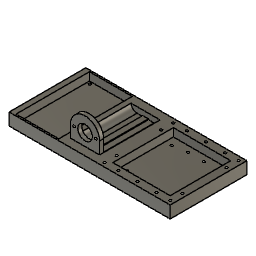
Base Péndulo v4 (Autodesk Fusion 360 design; units mm, degrees)
Autodesk Fusion 360 part; units mm, degrees
note: some values were not read from the file. Set by a fixed rule: which sketch regions a step uses.
sketch "Boceto1" plane through (0, 0, 0) normal (0, 0, 1) x (1, 0, 0)
  line L0 (0, 0) -> (0, 75)
  line L1 (0, 75) -> (71, 75)
  line L2 (71, 75) -> (71, 0)
  line L3 (71, 0) -> (0, 0)
  line L4 (71, 75) -> (81, 75)
  line L5 (81, 75) -> (81, 85)
  line L6 (81, 85) -> (-10, 85)
  line L7 (-10, 85) -> (-10, -10)
  line L8 (-10, -10) -> (81, -10)
  line L9 (81, -10) -> (81, 75)
  dimension "d1" = 75
  dimension "d2" = 71
  dimension "d3" = 10
  constraint coincident L0.start L3.end
  constraint vertical L0
  constraint perpendicular L0 L1
  constraint perpendicular L1 L2
  constraint perpendicular L0 L3
  constraint perpendicular L2 L4
  constraint perpendicular L4 L5
  constraint perpendicular L5 L6
  constraint perpendicular L6 L7
  constraint perpendicular L0 L8
  constraint perpendicular L4 L9
  measures "d1" distance of L0.start L0.end
  measures "d2" distance of L0.end L1.end
  measures "d3" distance of L1.end L4.end
extrude "Extruir1" add sketch "Boceto1" against normal blind 5 contours L0 L1 L2 L3 | L5 L6 L7 L8 L9 makes body 1
extrude "Extruir2" add sketch "Boceto1" along normal blind 10 bodies 1
sketch "Boceto2" plane through (0, 0, 0) normal (0, 0, 1) x (-1, 0, 0)
  line L0 (-71, -75) -> (0, -75)
  line L1 (0, -75) -> (0, 0)
  line L2 (0, 0) -> (-71, 0)
  line L3 (-71, 0) -> (-71, -75)
  line L4 (-35.5, -75) -> (-70.5, -75)
  line L5 (-35.5, -75) -> (-0.5, -75)
  line L6 (-0.5, -75) -> (-0.5, -55)
  line L7 (-0.5, -55) -> (-70.5, -55)
  line L8 (-70.5, -55) -> (-70.5, -75)
  line L9 (-0.5, -55) -> (-15.5, -55)
  line L10 (-15.5, -55) -> (-15.5, -75)
  line L11 (-70.5, -55) -> (-55.5, -55)
  line L12 (-55.5, -55) -> (-55.5, -75)
  line L13 (-15.5, -55) -> (-0.5, -75)
  line L14 (-55.5, -55) -> (-70.5, -75)
  line L15 (-15.5, -75) -> (-15.5, -60)
  line L16 (-15.5, -60) -> (-55.5, -60)
  line L17 (-35.5, -60) -> (-35.5, -75)
  line L18 (-35.5, -67.5) -> (-15.5, -67.5)
  line L19 (-35.5, -67.5) -> (-55.5, -67.5)
  circle A0 centre (-25.5, -67.5) radius 1.5
  circle A1 centre (-45.5, -67.5) radius 1.5
  circle A2 centre (-8, -65) radius 1.5
  circle A3 centre (-63, -65) radius 1.5
  dimension "d8" = 35
  dimension "d9" = 35
  dimension "d10" = 20
  dimension "d11" = 15
  dimension "d12" = 20
  dimension "d13" = 15
  dimension "d14" = 20
  dimension "d15" = 15
  dimension "d16" = 3
  dimension "d17" = 3
  dimension "d18" = 3
  dimension "d19" = 3
  constraint midpoint L0 L4.start
  constraint parallel L0 L4
  constraint parallel L0 L5
  constraint perpendicular L5 L6
  constraint perpendicular L3 L7
  constraint perpendicular L4 L8
  constraint perpendicular L6 L9
  constraint perpendicular L5 L10
  constraint perpendicular L8 L11
  constraint perpendicular L4 L12
  constraint perpendicular L5 L15
  constraint coincident L12 L16.end
  constraint perpendicular L12 L16
  constraint midpoint L16 L17.start
  constraint midpoint L17 L18.start
  constraint midpoint L15 L18.end
  constraint coincident L12 L19.end
  constraint perpendicular L12 L19
  constraint midpoint L18 A0.centre
  constraint midpoint L19 A1.centre
  constraint midpoint L13 A2.centre
  constraint midpoint L14 A3.centre
  measures "d8" distance of L4.start L4.end
  measures "d9" distance of L4.start L5.end
  measures "d10" distance of L5.end L6.end
  measures "d11" distance of L6.end L9.end
  measures "d12" distance of L9.end L10.end
  measures "d13" distance of L7.end L11.end
  measures "d14" distance of L11.end L12.end
  measures "d15" distance of L10.end L15.end
  measures "d16" diameter of A0
  measures "d17" diameter of A1
  measures "d18" diameter of A2
  measures "d19" diameter of A3
extrude "Extruir3" cut sketch "Boceto2" against normal up to surface (5 mm away) contours L14 A3 | L14 A3 | L19 A1 | L19 A1 | L18 A0 | L18 A0 | L13 A2 | L13 A2 bodies 1
sketch "Boceto3" plane through (0, 0, 10) normal (0, 0, 1) x (-1, 0, 0)
  line L0 (-71, -75) -> (-71, 0)
  line L1 (-71, 0) -> (0, 0)
  line L2 (0, 0) -> (0, -75)
  line L3 (0, -75) -> (-71, -75)
  line L4 (-81, 10) -> (-81, -85)
  line L5 (-81, -85) -> (10, -85)
  line L6 (10, -85) -> (10, 10)
  line L7 (10, 10) -> (-81, 10)
  line L8 (-71, -75) -> (-71, -60)
  line L9 (-71, -60) -> (-81, -60)
  line L10 (-81, -60) -> (-81, -85)
  line L11 (-81, -85) -> (10, -85)
  line L12 (0, -75) -> (0, -60)
  line L13 (0, -60) -> (10, -60)
  line L14 (10, -60) -> (10, -85)
  line L15 (0, -75) -> (-71, -75)
  line L16 (0, -75) -> (10, -75)
  line L17 (0, -75) -> (0, -85)
  line L18 (-71, -75) -> (-71, -85)
  line L19 (-71, -75) -> (-81, -75)
  circle A0 centre (5, -80) radius 1.5
  circle A1 centre (-76, -80) radius 1.5
  line L20 (10, -60) -> (0, -70)
  circle A2 centre (5, -65) radius 1.5
  line L21 (-81, -60) -> (-71, -70)
  circle A3 centre (-76, -65) radius 1.5
  line L22 (0, -85) -> (-23.6667, -85)
  line L23 (-71, -85) -> (-47.3333, -85)
  line L24 (-47.3333, -85) -> (-47.3333, -75)
  line L25 (-23.6667, -85) -> (-23.6667, -75)
  line L26 (-23.6667, -85) -> (0, -75)
  line L27 (-23.6667, -85) -> (-47.3333, -75)
  line L28 (-47.3333, -75) -> (-71, -85)
  circle A4 centre (-11.8333, -80) radius 1.5
  circle A5 centre (-35.5, -80) radius 1.5
  circle A6 centre (-59.1667, -80) radius 1.5
  dimension "d22" = 15
  dimension "d23" = 15
  dimension "d24" = 3
  dimension "d25" = 3
  dimension "d26" = 3
  dimension "d27" = 3
  dimension "d28" = 23.6667
  dimension "d29" = 23.6667
  dimension "d30" = 3
  dimension "d31" = 3
  dimension "d32" = 3
  constraint coincident L0.start L3.end
  constraint perpendicular L3 L8
  constraint coincident L4 L9.end
  constraint perpendicular L4 L9
  constraint coincident L4.end L5.start
  constraint coincident L5.end L6.start
  constraint coincident L2.end L3.start
  constraint perpendicular L3 L12
  constraint coincident L6 L13.end
  constraint perpendicular L6 L13
  constraint coincident L14 L16.end
  constraint coincident L5 L17.end
  constraint perpendicular L5 L17
  constraint perpendicular L15 L18
  constraint perpendicular L8 L19
  constraint midpoint L20 A2.centre
  constraint coincident L8 L21.end
  constraint midpoint L21 A3.centre
  constraint perpendicular L18 L22
  constraint perpendicular L18 L23
  constraint coincident L15 L24.end
  constraint perpendicular L15 L24
  constraint coincident L15 L25.end
  constraint perpendicular L15 L25
  constraint parallel L26 L28
  constraint midpoint L26 A4.centre
  constraint midpoint L27 A5.centre
  constraint midpoint L28 A6.centre
  measures "d22" distance of L0.start L8.end
  measures "d23" distance of L2.end L12.end
  measures "d24" diameter of A0
  measures "d25" diameter of A1
  measures "d26" diameter of A2
  measures "d27" diameter of A3
  measures "d28" distance of L17.end L22.end
  measures "d29" distance of L18.end L23.end
  measures "d30" diameter of A4
  measures "d31" diameter of A5
  measures "d32" diameter of A6
extrude "Extruir4" cut sketch "Boceto3" against normal up to surface (15 mm away) contours L21 A3 | L21 A3 | L27 A5 | L27 A5 | L28 A6 | L28 A6 | L26 A4 | L26 A4 | L20 A2 | L20 A2 | A0 | A1 bodies 1
ref_plane "PlanoDeObra1" through (35.5, 37.5, 2.5) normal (0, 1, 0) x (1, 0, 0)
split "Dividir1" by plane through (35.5, 37.5, 2.5) normal (0, 1, 0) bodies 1 makes body 2 at (32.2779, 47.0125, -5)
mirror "Simetría1" about plane through (35.5, 37.5, 2.5) normal (0, 1, 0) of bodies 2 merged
sketch "Boceto4" plane through (0, -10, 0) normal (0, -1, 0) x (1, 0, 0)
  line L0 (81, -5) -> (81, 10)
  line L1 (81, 10) -> (-10, 10)
  line L2 (-10, 10) -> (-10, -5)
  line L3 (-10, -5) -> (81, -5)
  line L4 (-10, -5) -> (81, -5)
  line L5 (35.5, -5) -> (-34.5, -5)
  line L6 (-34.5, -5) -> (-16.5, -5)
  line L7 (-34.5, -5) -> (-52.5, -5)
  line L8 (-16.5, -5) -> (-16.5, 10)
  line L9 (-16.5, 10) -> (-10, 10)
  line L10 (-52.5, -5) -> (-52.5, 25)
  line L11 (-16.5, -5) -> (-16.5, 25)
  line L12 (-16.5, 25) -> (-52.5, 25)
  circle A0 centre (-34.5, 25) radius 18
  circle A1 centre (-34.5, 25) radius 9
  line L13 (-34.5, 25) -> (-34.5, 3)
  line L14 (-34.5, 3) -> (-16.5, 3)
  line L15 (-34.5, 3) -> (-52.5, 3)
  line L16 (-52.5, -5) -> (-52.5, 10)
  line L17 (-52.5, 10) -> (-59, 10)
  line L18 (-59, 10) -> (-59, -5)
  line L19 (-59, -5) -> (-52.5, -5)
  line L20 (-43.5, 25) -> (-52.5, 25)
  line L21 (-25.5, 25) -> (-16.5, 25)
  circle A2 centre (-48, 25) radius 1.5
  circle A3 centre (-21, 25) radius 1.5
  dimension "d38" = 70
  dimension "d39" = 18
  dimension "d40" = 18
  dimension "d41" = 30
  dimension "d42" = 18
  dimension "d43" = 22
  dimension "d44" = 6.5
  dimension "d47" = 3
  dimension "d48" = 3
  constraint coincident L2.end L3.start
  constraint coincident L0.start L3.end
  constraint midpoint L4 L5.start
  constraint perpendicular L2 L5
  constraint parallel L5 L6
  constraint parallel L5 L7
  constraint perpendicular L1 L8
  constraint coincident L1.end L2.start
  constraint perpendicular L2 L9
  constraint perpendicular L7 L10
  constraint perpendicular L6 L11
  constraint midpoint L12 A0.centre
  constraint coincident L10.end A0
  constraint concentric A0 A1
  constraint coincident A0.centre A1.centre
  constraint perpendicular L12 L13
  constraint coincident L8 L14.end
  constraint coincident L10 L15.end
  constraint perpendicular L10 L15
  constraint midpoint L10 L16.end
  constraint perpendicular L16 L17
  constraint perpendicular L17 L18
  constraint coincident A1 L20.start
  constraint coincident L12 L20.start
  constraint coincident A1 L21.start
  constraint coincident L12 L21.start
  constraint midpoint L20 A2.centre
  constraint midpoint L21 A3.centre
  measures "d38" distance of L5.start L5.end
  measures "d39" distance of L5.end L6.end
  measures "d40" distance of L5.end L7.end
  measures "d41" distance of L7.end L10.end
  measures "d42" diameter of A1
  measures "d43" distance of A0.centre L13.end
  measures "d44" distance of L16.end L17.end
  measures "d47" diameter of A2
  measures "d48" diameter of A3
extrude "Extruir5" add sketch "Boceto4" against normal up to surface (95 mm away) contours L2 L5 L8 L9 L11 | L5 L6 L7 L8 L10 L11 L14 L15 L16 | L10 L16 L17 L18 L19 bodies 2
extrude "Extruir6" add sketch "Boceto4" against normal blind 5 contours L8 L11 A0 L13 L14 | L12 A0 A1 L13 L21 A3 | L12 A0 A1 L20 L21 A2 A3 | L10 A0 L13 L15 L16 | L12 A0 A1 L13 L20 A2 bodies 2
sketch "Boceto5" plane through (0, -5, 0) normal (0, 1, 0) x (-1, 0, 0)
  circle A0 centre (34.5, 25) radius 9
  circle A1 centre (48, 25) radius 1.5
  circle A2 centre (21, 25) radius 1.5
  line L0 (16.5, 25) -> (16.5, 10)
  line L1 (16.5, 10) -> (16.5, 3)
  line L2 (16.5, 3) -> (34.5, 3)
  line L3 (34.5, 3) -> (52.5, 3)
  line L4 (52.5, 3) -> (52.5, 10)
  line L5 (52.5, 10) -> (52.5, 25)
  arc A3 (52.5, 25) -> (16.5, 25) centre (34.5, 25) ccw
  line L6 (34.5, 3) -> (38, 3)
  line L7 (34.5, 3) -> (31, 3)
  line L8 (31, 3) -> (31, 4)
  line L9 (31, 4) -> (38, 4)
  line L10 (38, 4) -> (38, 3)
  dimension "d51" = 3.5
  dimension "d52" = 3.5
  constraint coincident L2.end L3.start
  constraint parallel L3 L6
  constraint parallel L2 L7
  constraint perpendicular L7 L8
  constraint perpendicular L8 L9
  measures "d51" distance of L2.end L6.end
  measures "d52" distance of L2.end L7.end
extrude "Extruir7" add sketch "Boceto5" along normal up to surface (90 mm away) contours L2 L3 L6 L7 L8 L9 L10 bodies 2
sketch "Boceto6" plane through (0, -5, 0) normal (0, 1, 0) x (-1, 0, 0)
  line L0 (31, 3) -> (31, 4)
  line L1 (31, 4) -> (38, 4)
  line L2 (38, 4) -> (38, 3)
  line L3 (38, 3) -> (52.5, 3)
  line L4 (52.5, 3) -> (52.5, 10)
  line L5 (52.5, 10) -> (52.5, 25)
  arc A0 (52.5, 25) -> (16.5, 25) centre (34.5, 25) ccw
  line L6 (16.5, 25) -> (16.5, 10)
  line L7 (16.5, 10) -> (16.5, 3)
  line L8 (16.5, 3) -> (31, 3)
  circle A1 centre (21, 25) radius 1.5
  circle A2 centre (48, 25) radius 1.5
  circle A3 centre (34.5, 25) radius 9
  circle A4 centre (34.5, 25) radius 22.5
  dimension "d55" = 45
  constraint concentric A0 A4
  measures "d55" diameter of A4
fillet "Empalme1" radius 7.5 2 edges at (-52.5, 40, 3) (-16.5, 40, 3) on bodies 2
sketch "Boceto7" plane through (0, 85, 0) normal (0, 1, 0) x (-1, 0, 0)
  line L0 (-81, 10) -> (-81, -5)
  line L1 (-81, -5) -> (52.5, -5)
  line L2 (52.5, -5) -> (59, -5)
  line L3 (59, -5) -> (59, 10)
  line L4 (59, 10) -> (52.5, 10)
  arc A0 (45.0167, 3) -> (52.5, 10) centre (45.0167, 10.5) ccw
  line L5 (45.0167, 3) -> (38, 3)
  line L6 (38, 3) -> (38, 4)
  line L7 (38, 4) -> (31, 4)
  line L8 (31, 4) -> (31, 3)
  line L9 (31, 3) -> (23.9833, 3)
  arc A1 (16.5, 10) -> (23.9833, 3) centre (23.9833, 10.5) ccw
  line L10 (16.5, 10) -> (-81, 10)
  line L11 (16.5, 10) -> (52.5, 10)
  constraint coincident A1.start L10.start
  constraint coincident L4.end A0.end
extrude "Extruir8" add sketch "Boceto7" against normal blind 20 contours A0 L5 L6 L7 L8 L9 A1 L11 bodies 2
sketch "Boceto8" plane through (0, -10, 0) normal (0, -1, 0) x (1, 0, 0)
  circle A0 centre (-21, 25) radius 1.5
  circle A1 centre (-48, 25) radius 1.5
  circle A2 centre (-34.5, 25) radius 9
  line L0 (81, -5) -> (81, 10)
  line L1 (81, 10) -> (-16.5, 10)
  line L2 (-16.5, 10) -> (-16.5, 25)
  arc A3 (-16.5, 25) -> (-52.5, 25) centre (-34.5, 25) ccw
  line L3 (-52.5, 25) -> (-52.5, 10)
  line L4 (-52.5, 10) -> (-59, 10)
  line L5 (-59, 10) -> (-59, -5)
  line L6 (-59, -5) -> (-52.5, -5)
  line L7 (-52.5, -5) -> (81, -5)
  line L8 (-59, 10) -> (-59, 0)
  line L9 (-59, 0) -> (-112, 0)
  line L10 (-112, 0) -> (-112, 10)
  line L11 (-112, 10) -> (-118.5, 10)
  line L12 (-59, -5) -> (-112, -5)
  line L13 (-112, -5) -> (-118.5, -5)
  line L14 (-118.5, -5) -> (-118.5, 10)
  dimension "d60" = 53
  dimension "d61" = 6.5
  constraint coincident L4.end L5.start
  constraint coincident L5 L8.end
  constraint perpendicular L4 L8
  constraint perpendicular L5 L9
  constraint perpendicular L9 L10
  constraint perpendicular L3 L11
  constraint coincident L5.end L6.start
  constraint perpendicular L5 L12
  constraint perpendicular L5 L13
  measures "d60" distance of L8.end L9.end
  measures "d61" distance of L10.end L11.end
extrude "Extruir9" add sketch "Boceto8" against normal up to surface (95 mm away) contours L5 L9 L10 L11 L12 L13 L14 bodies 2
sketch "Boceto9" plane through (0, -10, 0) normal (0, -1, 0) x (1, 0, 0)
  circle A0 centre (-21, 25) radius 1.5
  circle A1 centre (-48, 25) radius 1.5
  circle A2 centre (-34.5, 25) radius 9
  line L0 (81, -5) -> (81, 10)
  line L1 (81, 10) -> (-16.5, 10)
  line L2 (-16.5, 10) -> (-16.5, 25)
  arc A3 (-16.5, 25) -> (-52.5, 25) centre (-34.5, 25) ccw
  line L3 (-52.5, 25) -> (-52.5, 10)
  line L4 (-52.5, 10) -> (-59, 10)
  line L5 (-59, 10) -> (-59, 0)
  line L6 (-59, 0) -> (-112, 0)
  line L7 (-112, 0) -> (-112, 10)
  line L8 (-112, 10) -> (-118.5, 10)
  line L9 (-118.5, 10) -> (-118.5, -5)
  line L10 (-118.5, -5) -> (-112, -5)
  line L11 (-112, -5) -> (-59, -5)
  line L12 (-59, -5) -> (-52.5, -5)
  line L13 (-52.5, -5) -> (81, -5)
  line L14 (-112, 10) -> (-59, 10)
  constraint coincident L7.end L8.start
  constraint coincident L4.end L5.start
sketch "Boceto10" plane through (0, 85, 0) normal (0, 1, 0) x (-1, 0, 0)
  line L0 (-81, 10) -> (-81, -5)
  line L1 (-81, -5) -> (52.5, -5)
  line L2 (52.5, -5) -> (59, -5)
  line L3 (59, -5) -> (112, -5)
  line L4 (112, -5) -> (118.5, -5)
  line L5 (118.5, -5) -> (118.5, 10)
  line L6 (118.5, 10) -> (112, 10)
  line L7 (112, 10) -> (112, 0)
  line L8 (112, 0) -> (59, 0)
  line L9 (59, 0) -> (59, 10)
  line L10 (59, 10) -> (-81, 10)
  line L11 (59, 10) -> (112, 10)
  constraint coincident L9.end L10.start
  constraint coincident L6.end L7.start
extrude "Extruir10" add sketch "Boceto10" against normal blind 2 contours L7 L8 L9 L11 bodies 2
extrude "Extruir11" add sketch "Boceto9" against normal blind 2 contours L5 L6 L7 L14 bodies 2
sketch "Boceto11" plane through (0, 0, 0) normal (0, 0, 1) x (-1, 0, 0)
  line L0 (112, 8) -> (59, 8)
  line L1 (59, 8) -> (59, -83)
  line L2 (59, -83) -> (112, -83)
  line L3 (112, -83) -> (112, 8)
  line L4 (59, -83) -> (59, -82.5)
  line L5 (59, -82.5) -> (112, -82.5)
  line L6 (59, 8) -> (59, 7.5)
  line L7 (59, 7.5) -> (112, 7.5)
  line L8 (112, 7.5) -> (111, 7.5)
  line L9 (111, 7.5) -> (111, -82.5)
  line L10 (59, -82.5) -> (60, -82.5)
  line L11 (60, -82.5) -> (60, 7.5)
  line L12 (111, 7.5) -> (111, 6.5)
  line L13 (111, 6.5) -> (110, 6.5)
  line L14 (110, 6.5) -> (60, 6.5)
  line L15 (60, 7.5) -> (61, 7.5)
  line L16 (61, 7.5) -> (61, -82.5)
  line L17 (60, -82.5) -> (60, -81.5)
  line L18 (60, -81.5) -> (111, -81.5)
  line L19 (111, -82.5) -> (110, -82.5)
  line L20 (110, -82.5) -> (110, 6.5)
  circle A0 centre (108.5, 5) radius 1.5
  circle A1 centre (62.5, 5) radius 1.5
  circle A2 centre (108.5, -80) radius 1.5
  circle A3 centre (62.5, -80) radius 1.5
  dimension "d68" = 0.5
  dimension "d69" = 53
  dimension "d70" = 0.5
  dimension "d71" = 53
  dimension "d72" = 1.5
  dimension "d73" = 1.5
  dimension "d74" = 1.5
  dimension "d75" = 1.5
  constraint coincident L1.end L2.start
  constraint perpendicular L2 L4
  constraint perpendicular L1 L5
  constraint coincident L0.end L1.start
  constraint perpendicular L0 L6
  constraint perpendicular L1 L7
  constraint coincident L7 L8.end
  constraint coincident L5 L9.end
  constraint perpendicular L5 L9
  constraint coincident L5 L10.end
  constraint coincident L7 L11.end
  constraint perpendicular L7 L11
  constraint coincident L9 L12.end
  constraint perpendicular L9 L13
  constraint coincident L11 L14.end
  constraint perpendicular L11 L14
  constraint coincident L7 L15.end
  constraint coincident L5 L16.end
  constraint perpendicular L5 L16
  constraint coincident L11 L17.end
  constraint coincident L9 L18.end
  constraint perpendicular L9 L18
  constraint coincident L5 L19.end
  constraint perpendicular L14 L20
  constraint tangent L20 A0
  constraint tangent L14 A0
  constraint tangent L16 A1
  constraint tangent L14 A1
  constraint tangent L18 A2
  constraint tangent L20 A2
  constraint tangent L18 A3
  constraint tangent L16 A3
  measures "d68" distance of L1.end L4.end
  measures "d69" distance of L4.end L5.end
  measures "d70" distance of L0.end L6.end
  measures "d71" distance of L6.end L7.end
  measures "d72" radius of A0
  measures "d73" radius of A1
  measures "d74" radius of A2
  measures "d75" radius of A3
extrude "Extruir12" cut sketch "Boceto11" against normal up to surface (5 mm away) contours A1 | A0 | A2 | A3 bodies 2
extrude "Extruir13" cut 1 faces at (-33.3333, 65, 8) along direction (0, 1, 0) blind 10 on bodies 2 bodies 2
extrude "Extruir14" add 1 faces at (-23.124, -5, 10.3212) along direction (0, 1, 0) blind 10 on bodies 2 bodies 2
sketch "Boceto12" plane through (0, -10, 0) normal (0, -1, 0) x (1, 0, 0)
  circle A0 centre (-21, 25) radius 1.5
  circle A1 centre (-48, 25) radius 1.5
  circle A2 centre (-34.5, 25) radius 9
  line L0 (81, -5) -> (81, 10)
  line L1 (81, 10) -> (-16.5, 10)
  line L2 (-16.5, 10) -> (-16.5, 25)
  arc A3 (-16.5, 25) -> (-52.5, 25) centre (-34.5, 25) ccw
  line L3 (-52.5, 25) -> (-52.5, 10)
  line L4 (-52.5, 10) -> (-118.5, 10)
  line L5 (-118.5, 10) -> (-118.5, -5)
  line L6 (-118.5, -5) -> (-112, -5)
  line L7 (-112, -5) -> (-59, -5)
  line L8 (-59, -5) -> (-52.5, -5)
  line L9 (-52.5, -5) -> (81, -5)
  line L10 (-52.5, 10) -> (-16.5, 10)
  constraint coincident L3.end L4.start
  constraint coincident L1.end L2.start
extrude "Extruir15" cut sketch "Boceto12" against normal blind 10 contours L2 A3 L3 L10 bodies 2
hidden bodies 1
equation "d28 = ( 71 / 3 ) * 1 mm"
equation "d29 = ( 71 / 3 ) * 1 mm"
equation "d35 = ( -95 / 2 ) * 1 mm"
equation "d43 = 9 mm + 13 mm"
